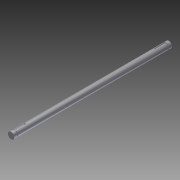
# Autodesk Inventor part: 8 ball roller shaft
Saved by Autodesk Inventor 2012 (Build 160160000, 160)
## iProperties
Created: 2013-11-12
Part Number: 8 ball roller shaft
Material: Default
Document SubType Name: Modeling
Designer: Bryce
Density: 1 g/cm^3
Author: Bryce
Autodesk Inventor part; units mm, degrees
sketch "Sketch1" plane through (0, 0, 0) normal (0, 0, 1) x (1, 0, 0)
  circle A0 centre (0, 0) radius 6.35
  dimension "d0" = 12.7
  constraints: 1 centre point, 1 coincident
  measures "d0" diameter of A0
extrude "Extrusion1" add sketch "Sketch1" along normal blind 314.325
ref_plane "Work Plane1" through (0, 6.35, 0) normal (0, 1, 0) x (-1, 0, 0)
sketch "Sketch2" plane through (0, 6.35, 0) normal (0, 1, 0) x (-1, 0, 0)
  line L0 (-6.35, 314.325) -> (6.35, 314.325) projected
  line L1 (-6.35, 0) -> (6.35, 0) projected
  line L2 (-6.35, 0) -> (-6.35, 314.325) projected
  line L3 (6.35, 0) -> (6.35, 314.325) projected
  line L4 (-6.35, 6.35) -> (6.35, 6.35)
  line L5 (-6.35, 307.975) -> (6.35, 307.975)
  arc A0 (1.5875, 306.3875) -> (-1.5875, 306.3875) centre (0, 306.3875) ccw
  line L6 (-1.5875, 306.3875) -> (-1.5875, 287.3375)
  line L7 (1.5875, 306.3875) -> (1.5875, 287.3375)
  arc A1 (-1.5875, 287.3375) -> (1.5875, 287.3375) centre (0, 287.3375) ccw
  arc A2 (1.5875, 26.9875) -> (-1.5875, 26.9875) centre (0, 26.9875) ccw
  line L8 (-1.5875, 26.9875) -> (-1.5875, 7.9375)
  line L9 (1.5875, 26.9875) -> (1.5875, 7.9375)
  arc A3 (-1.5875, 7.9375) -> (1.5875, 7.9375) centre (0, 7.9375) ccw
  point P0 (0, 0)
  dimension "d3" = 301.625
  dimension "d4" = 6.35
  dimension "d5" = 6.35
  dimension "d11" = 19.05
  dimension "d12" = 3.175
  dimension "d13" = 19.05
  dimension "d14" = 3.175
  dimension "d15" = 7.9375
  dimension "d16" = 279.4
  dimension "d17" = 6.35
  constraints: 12 end point, 8 point on circle, 6 tangent, 4 centre point, 4 point on line, 3 perpendicular, 3 vertical alignment, 2 equal radius, 2 parallel
  measures "d3" distance between parallel lines of L4 L5
  measures "d4" distance between parallel lines of L1 L4
  measures "d5" distance between parallel lines of L0 L5
  measures "d11" distance of A1.centre A0.centre
  measures "d12" distance between parallel lines of L7 L6
  measures "d13" distance of A3.centre A2.centre
  measures "d14" distance between parallel lines of L9 L8
  measures "d15" distance from line of L0 A0.centre
  measures "d16" distance of A3.centre A1.centre
  measures "d17" distance from line of L2 A0.centre
ref_plane "Work Plane2" through (6.35, 6.35, 307.975) normal (0, 0, 1) x (1, 0, 0)
ref_plane "Work Plane3" through (6.35, 6.35, 6.35) normal (0, 0, -1) x (-1, 0, 0)
sketch "Sketch3" plane through (6.35, 6.35, 307.975) normal (0, 0, 1) x (1, 0, 0)
  circle A0 centre (-6.35, -6.35) radius 6.35 projected
  circle A1 centre (-6.35, -6.35) radius 5.08
  dimension "d6" = 10.16
  constraints: 1 centre point, 1 coincident
  measures "d6" diameter of A1
extrude "Extrusion2" cut sketch "Sketch3" against normal blind 1.016
sketch "Sketch4" plane through (6.35, 6.35, 6.35) normal (0, 0, -1) x (-1, 0, 0)
  circle A0 centre (6.35, -6.35) radius 5.08 projected
  circle A1 centre (6.35, -6.35) radius 6.35 projected
extrude "Extrusion3" cut sketch "Sketch4" against normal blind 1.016
extrude "Extrusion4" cut sketch "Sketch2" against normal blind 1.5875 contours A3 L8 A2 L9 | A0 L7 A1 L6
equation "\"d4\" = d5"
body "Solid1"
